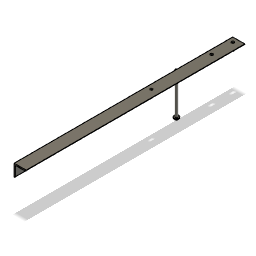
Equerre-Gauche 80x80x8 longueur 1450mm (Autodesk Fusion 360 design; units mm, degrees)
Autodesk Fusion 360 part; units mm, degrees
note: some values were not read from the file. Set by a fixed rule: which sketch regions a step uses.
sketch "Sketch1" plane through (0, 0, 0) normal (0, 0, 1) x (1, 0, 0)
  line L0 (0, 0) -> (0, 80)
  line L1 (0, 80) -> (80, 80)
  line L2 (8, 6) -> (8, 68)
  line L3 (12, 72) -> (74, 72)
  line L4 (80, 78) -> (80, 80)
  line L5 (0, 0) -> (2, 0)
  arc A0 (74, 72) -> (80, 78) centre (74, 78) ccw
  arc A1 (2, 0) -> (8, 6) centre (2, 6) ccw
  arc A2 (12, 72) -> (8, 68) centre (12, 68) ccw
  dimension "d1" = 80
  dimension "d2" = 80
  dimension "d4" = 6
  dimension "d5" = 6
  dimension "d6" = 4
  constraint coincident L0.start L5.start
  constraint horizontal L1
  constraint vertical L0
  constraint perpendicular L1 L4
  constraint perpendicular L2 L5
  constraint parallel L0 L2
  constraint parallel L1 L3
  constraint tangent L3 A0
  constraint tangent L4 A0
  constraint tangent L2 A1
  constraint tangent L5 A1
  constraint tangent L2 A2
  constraint tangent L3 A2
  measures "d1" distance of L0.start L0.end
  measures "d2" distance of L0.end L1.end
  measures "d4" radius of A0
  measures "d5" radius of A1
  measures "d6" radius of A2
extrude "Extrude1" add sketch "Sketch1" along normal mid plane 1450
sketch "Sketch4" plane through (0, 0, 0) normal (-1, 0, 0) x (0, 0, 1)
  line L0 (-725, 0) -> (725, 0) construction
  line L1 (725, 0) -> (725, 80) construction
  line L2 (725, 80) -> (-725, 80) construction
  line L3 (-725, 80) -> (-725, 0) construction
  line L4 (-725, 0) -> (725, 0) construction
  line L5 (-725, 80) -> (725, 80) construction
  line L6 (-725, 0) -> (-725, 80) construction
  line L7 (725, 80) -> (725, 0) construction
  line L8 (0, 0) -> (0, 80) construction
  line L9 (-725, 40) -> (725, 40) construction
  line L10 (-725, 80) -> (-725, -420) construction
  line L11 (285, 80) -> (285, -420) construction
  line L12 (365, 80) -> (365, -420) construction
  line L13 (425, 80) -> (425, -420) construction
  line L14 (620, 80) -> (620, -420) construction
  line L15 (690, 80) -> (690, -420) construction
  line L16 (629, 31) -> (681, 31)
  arc A0 (681, 31) -> (681, 49) centre (681, 40) ccw
  line L17 (681, 49) -> (629, 49)
  arc A1 (629, 49) -> (629, 31) centre (629, 40) ccw
  line L18 (620, 40) -> (690, 40) construction
  circle A2 centre (285, 40) radius 9
  circle A3 centre (365, 40) radius 9
  circle A4 centre (425, 40) radius 9
  dimension "d16" = 1010
  dimension "d17" = 1090
  dimension "d18" = 1150
  dimension "d19" = 1345
  dimension "d20" = 1415
  dimension "d21" = 18
  dimension "d22" = 18
  dimension "d23" = 18
  dimension "d24" = 18
  constraint coincident L8.start origin
  constraint midpoint L2 L8.end
  constraint midpoint L3 L9.start
  constraint midpoint L7 L9.end
  constraint coincident L2.end L3.start
  constraint vertical L10
  constraint tangent L16 A0
  constraint tangent A0 L17
  constraint parallel L16 L17
  constraint tangent L17 A1
  constraint tangent L16 A1
  constraint midpoint A1 L18.start
  constraint midpoint A0 L18.end
  constraint coincident L9 L18.end
  constraint coincident L15 L18.end
  constraint perpendicular L15 L18
  constraint coincident L9 L18.start
  constraint coincident L14 L18.start
  constraint coincident L11 A2.centre
  constraint coincident L9 A2.centre
  constraint coincident L12 A3.centre
  constraint coincident L9 A3.centre
  constraint coincident L13 A4.centre
  constraint coincident L9 A4.centre
  measures "d21" diameter of A0
  measures "d22" diameter of A2
  measures "d23" diameter of A3
  measures "d24" diameter of A4
extrude "Extrude4" cut sketch "Sketch4" against normal through all
sketch "Sketch5" plane through (0, 80, 0) normal (0, 1, 0) x (-1, 0, 0)
  line L0 (0, -725) -> (0, 725) construction
  line L1 (0, 725) -> (-80, 725)
  line L2 (-80, 725) -> (-80, -725) construction
  line L3 (-80, -725) -> (0, -725) construction
  line L4 (-80, -725) -> (-80, 725) construction
  line L5 (0, -725) -> (-80, -725) construction
  line L6 (0, -725) -> (0, 725) construction
  line L7 (-30, -725) -> (-30, 725) construction
  line L8 (-80, -725) -> (384.3429, -725) construction
  line L9 (-80, -695) -> (384.3429, -695) construction
  line L10 (-80, -555) -> (384.3429, -555) construction
  line L11 (-80, -155) -> (384.3429, -155) construction
  circle A0 centre (-30, -695) radius 9
  circle A1 centre (-30, -555) radius 9
  circle A2 centre (-30, -155) radius 8
  dimension "d26" = 30
  dimension "d27" = 30
  dimension "d28" = 170
  dimension "d29" = 570
  dimension "d30" = 18
  dimension "d31" = 18
  dimension "d32" = 16
  constraint coincident L2.end L3.start
  constraint perpendicular L4 L8
  constraint coincident L9 A0.centre
  constraint coincident L7 A0.centre
  constraint coincident L10 A1.centre
  constraint coincident L7 A1.centre
  constraint coincident L11 A2.centre
  constraint coincident L7 A2.centre
  measures "d30" diameter of A0
  measures "d31" diameter of A1
  measures "d32" diameter of A2
extrude "Extrude5" cut sketch "Sketch5" against normal through all
ref_plane "WorkPlane1" through (40, 74, 0) normal (0, 1, 0) x (-1, 0, 0)
sketch "Sketch6" plane through (40, 74, 0) normal (0, 1, 0) x (1, 0, 0)
  line L0 (-40, 725) -> (-40, -725) construction
  line L1 (-40, 725) -> (40, 725) construction
  line L2 (40, 725) -> (40, -725) construction
  line L3 (40, 725) -> (-288.3779, 725)
  line L4 (40, 355) -> (-288.3779, 355)
  line L5 (-43.5, 725) -> (-43.5, -725) construction
  circle A0 centre (-43.5, 355) radius 8
  dimension "d35" = 370
  dimension "d36" = 3.5
  dimension "d37" = 16
  constraint coincident L1.end L2.start
  constraint perpendicular L2 L3
  constraint coincident L4 A0.centre
  constraint coincident L5 A0.centre
  measures "d37" diameter of A0
extrude "Extrude6" add sketch "Sketch6" against normal blind 284
ref_plane "WorkPlane2" through (-3.5, -200, -355) normal (0, -1, 0) x (-1, 0, 0)
sketch "Sketch7" plane through (-3.5, -200, -355) normal (0, -1, 0) x (1, 0, 0)
  circle A0 centre (0, 0) radius 16
  dimension "d41" = 32
  constraint coincident A0.centre origin
  measures "d41" diameter of A0
extrude "Extrude7" add sketch "Sketch7" against normal blind 5
chamfer "Chamfer1" distance 1 angle 45 1 edges at (-10.9586, -210, -357.8929)
